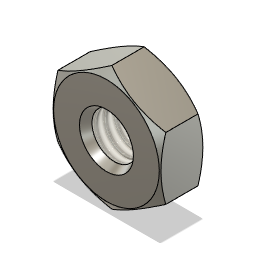
Support for Capacitor Board (Autodesk Fusion 360 archive; units mm, degrees)
design "Hexagon Nut DIN 934 - M2.5 x 0.45 Steel 6 Plain"
description: Hexagon Nut DIN 934 - M2.5 x 0.45
Autodesk Fusion 360 part; units mm, degrees
sketch "Sketch1" plane through (0, 0, 0) normal (0, 1, 0) x (1, 0, 0)
  line L0 (0, 0) -> (0, -2)
  line L1 (-1.25, 0) -> (-2.45, 0)
  line L2 (-2.45, 0) -> (-2.8875, -0.2526)
  line L3 (-2.8875, -0.2526) -> (-2.8875, -1.7474)
  line L4 (-2.8875, -1.7474) -> (-2.45, -2)
  line L5 (-2.45, -2) -> (-1.25, -2)
  line L6 (-1.25, -2) -> (-1.25, 0)
  dimension "d121" = 2.5
  dimension "d122" = 30
  dimension "d123" = 30
  dimension "d126" = 2
  dimension "d128" = 5.775
  dimension "d172" = 4.9
  constraint vertical L0
  constraint coincident L0 L0.end
  constraint coincident origin L0
  constraint horizontal L1
  constraint perpendicular L1 L3
  constraint perpendicular L3 L5
  constraint perpendicular L5 L6
  constraint coincident L0.start L1
  constraint coincident L0.start origin
  constraint coincident L0.end L5
  constraint equal L1 L5
  measures "d122" angle of L1 L2
  measures "d123" angle of L4 L5
  measures "d126" distance of L1.start L5.end
revolve "Revolve1" add sketch "Sketch1" angle 360 about axis through (0, 0, 0) along (0, 0, 1)
sketch "Sketch8" plane through (0, 0, 2) normal (0, 0, 1) x (1, 0, 0)
  line L0 (0, 0) -> (-5, 0) construction
  line L1 (-2.5, -1.4449) -> (-2.5, 1.4449)
  circle A0 centre (0, 0) radius 1.25
  circle A1 centre (0, 0) radius 2.8875
  dimension "d114" = 2.5
  constraint horizontal L0
  constraint perpendicular L0 L1
  constraint midpoint L0 L1
  constraint coincident L0.start A0.centre
  constraint coincident L1.end A1
  measures "d114" distance of L0.start L1
extrude "Extrude5" cut sketch "Sketch8" against normal blind 2 contours L1 A1 picked at (-2.5625, 0.3519)
pattern_circular "C-Pattern2" count 6 over 360 about axis through (0, 0, 1.75) along (0, 0, 1) of "Extrude5"
thread "Thread3" "ISO Metric profile 2.5 M2.5x0.45 6H" major diameter 2.58 minor diameter 2.0755 pitch 0.45 angle 60 resizes the face on face at (-1.2438, 0.1245, 1.3333)
sketch "Sketch12" plane through (0, 0, 0) normal (0, 1, 0) x (1, 0, 0)
  line L0 (1.0377, -2) -> (-1.0377, -2)
  line L1 (2.45, -2) -> (-2.45, -2)
  line L2 (2.45, 0) -> (-2.45, 0)
  line L3 (1.0377, 0) -> (-1.0377, 0)
  line L4 (-1.25, 0) -> (0, 0)
  line L5 (-0.6726, -1) -> (-1.25, 0)
  line L6 (-1.25, -2) -> (0, -2)
  line L7 (-0.6726, -1) -> (-1.25, -2)
  line L8 (0, 0) -> (0, -2)
  dimension "d165" = 60
  dimension "d169" = 60
  dimension "d170" = 1.25
  constraint horizontal L4
  constraint collinear L1 L6
  constraint coincident L5.start L7.start
  constraint vertical L4.start L6.start
  constraint coincident L1 L6.end
  constraint coincident L6.end L8.end
  constraint coincident L4.end L8.start
  measures "d165" angle of L2 L5
  measures "d169" angle of L6 L7
  measures "d170" distance of L4.start L4.end
revolve "Revolve3" cut sketch "Sketch12" angle 360 about axis through (0, 0, 1.75) along (0, 0, 1)
equation "adsk_nheig = 2.00 mm"
equation "adsk_maxdia = 5.775 mm"
equation "adsk_nomdia = 2.50 mm"
equation "d89 = -adsk_nheig"
equation "adsk_waflat = 5.00 mm"
equation "d114 = adsk_waflat / 2"
equation "adsk_chamang1 = 30.00 deg"
equation "adsk_chamang2 = 30.00 deg"
equation "d121 = adsk_nomdia"
equation "d122 = adsk_chamang1"
equation "d123 = adsk_chamang2"
equation "d126 = adsk_nheig"
equation "d128 = adsk_maxdia"
equation "d163 = adsk_nheig"
equation "d170 = adsk_nomdia * 0.5"
equation "adsk_beardia = adsk_waflat * 0.98"
equation "d172 = adsk_beardia"
